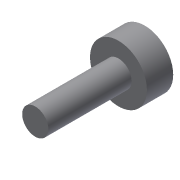
# Autodesk Inventor part: HeightScrew
Saved by Autodesk Inventor 2014 (Build 180170000, 170)
## iProperties
Created: 2014-09-08
Part Number: HeightScrew
Material: Generic
Document SubType Name: Modeling
Designer: Peele
Density: 1 g/cm^3
Appearance: Default
Author: Peele
Autodesk Inventor part; units mm, degrees
ref_plane "YZ Plane" through (0, 0, 0) normal (1, 0, 0) x (0, 1, 0)
ref_plane "XZ Plane" through (0, 0, 0) normal (0, 1, 0) x (-1, 0, 0)
ref_plane "XY Plane" through (0, 0, 0) normal (0, 0, 1) x (1, 0, 0)
sketch "Sketch1" plane through (0, 0, 0) normal (0, 0, 1) x (1, 0, 0)
  line L0 (0, 0) -> (0, -25)
  line L1 (0, -25) -> (3, -25)
  line L2 (3, -25) -> (3, -6)
  line L3 (3, -6) -> (6.5, -6)
  line L4 (6.5, -6) -> (6.5, 0)
  line L5 (6.5, 0) -> (0, 0)
  dimension "d0" = 19
  dimension "d1" = 6
  dimension "d2" = 6.5
  dimension "d3" = 3
  constraints: 12 end point, 4 parallel, 1 perpendicular, 1 vertical
  measures "d0" distance of L1.end L2.end
  measures "d1" distance of L3.end L4.end
  measures "d2" distance of L4.end L0.start
  measures "d3" distance of L0.end L1.end
revolve "Revolution1" add sketch "Sketch1" angle 360 about axis through (0, 0, 0) along (0, -1, 0)
body "Solid1"
